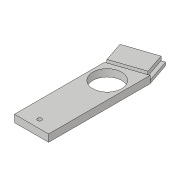
# Autodesk Inventor part: Lidar Sensor Case Piece 2
Saved by Autodesk Inventor 2018.3 (Build 223284000, 284)
## iProperties
Created: 2019-02-26
Part Number: Lidar Sensor Case Piece 2
Material: Generic
Document SubType Name: Modeling
Designer: aye06091
Mass: 11.3761 g
Surface Area: 61.4411 cm^2
Volume: 11.3761 cm^3
Density: 1 g/cm^3
Appearance: Default
Author: aye06091
Autodesk Inventor part; units mm, degrees
ref_plane "YZ Plane" through (0, 0, 0) normal (1, 0, 0) x (0, 1, 0)
ref_plane "XZ Plane" through (0, 0, 0) normal (0, 1, 0) x (-1, 0, 0)
ref_plane "XY Plane" through (0, 0, 0) normal (0, 0, 1) x (1, 0, 0)
sketch "Sketch1" plane through (0, 0, 0) normal (0, 1, 0) x (-1, 0, 0)
  line L0 (18.6455, 5.0782) -> (18.6456, 5.0782)
  line L1 (-34.5212, -28.5033) -> (-28.4641, -46.5646)
  line L2 (-28.4641, -46.5646) -> (-1.974, -37.6808)
  circle A0 centre (-21.2762, -8.5069) radius 11.176
  line L3 (-8.0312, 50.2306) -> (-8.0312, -19.6194)
  line L4 (-8.0312, -19.6194) -> (-1.974, -37.6808)
  line L5 (-1.974, -37.6808) -> (-28.4641, -46.5646)
  line L6 (-28.4641, -46.5646) -> (-34.5212, -28.5033)
  line L7 (-34.5212, -28.5033) -> (-34.5212, 50.2306)
  line L8 (-8.0312, 50.2306) -> (-34.5212, 50.2306)
  point P0 (0, 0)
  dimension "d2" = 27.94
  dimension "d4" = 22.352
  dimension "d24" = 19.05
  dimension "d25" = 69.85
  dimension "d26" = 19.05
  dimension "d28" = 26.49
  dimension "d29" = 13.245
  dimension "d35" = 58.7375
  constraints: 18 end point, 4 perpendicular, 1 centre point, 1 parallel, 1 vertical
  measures "d2" distance of L1.end L2.end
  measures "d4" diameter of A0
  measures "d24" distance of L3.end L2.end
  measures "d25" distance of L3.start L3.end
  measures "d26" distance of L1.start L1.end
  measures "d28" distance of L3.start L7.end
  measures "d29" distance from line of L7 A0.centre
  measures "d35" distance from line of L8 A0.centre
extrude "Extrusion1" add sketch "Sketch1" along normal blind 5.6134
sketch "Sketch2" plane through (0, 5.6134, 0) normal (0, 1, 0) x (1, 0, 0)
  line L0 (34.5212, 28.5034) -> (8.0312, 19.6194)
  line L1 (8.0312, 19.6194) -> (7.0701, 22.4851)
  line L2 (7.0701, 22.4851) -> (33.5601, 31.3691)
  line L3 (31.5176, 27.4961) -> (29.9884, 26.9832)
  line L4 (34.5212, 28.5033) -> (28.4641, 46.5646) projected
  point P0 (0, 0)
  point P1 (0, 0)
  dimension "d11" = 3.0226
  constraints: 8 end point, 4 point on line, 1 parallel, 1 perpendicular
  measures "d11" distance between parallel lines of L2 L0
extrude "Extrusion2" cut sketch "Sketch2" against normal blind 3.175
sketch "Sketch3" plane through (0, 5.6134, 0) normal (0, 1, 0) x (1, 0, 0)
  line L0 (7.0701, 22.4852) -> (33.5601, 31.3691) projected
  line L1 (33.5601, 31.3691) -> (28.4641, 46.5646) projected
  line L2 (28.4641, 46.5646) -> (1.974, 37.6808) projected
  line L3 (25.803, 45.6722) -> (30.8991, 30.4767)
  point P0 (0, 0)
  dimension "d17" = 2.8067
  constraints: 2 end point, 2 point on line, 1 parallel
  measures "d17" distance between parallel lines of L1 L3
extrude "Extrusion3" cut sketch "Sketch3" against normal blind 3.175
sketch "Sketch4" plane through (0, 5.6134, 0) normal (0, 1, 0) x (1, 0, 0)
  line L0 (8.0312, -50.2306) -> (34.5212, -50.2306) projected
  line L1 (34.5212, -50.2306) -> (34.5212, 28.5033) projected
  circle A0 centre (21.2762, -43.8806) radius 1.6002
  point P0 (0, 0)
  dimension "d30" = 3.2004
  dimension "d31" = 13.245
  dimension "d32" = 6.35
  constraints: 1 centre point
  measures "d30" diameter of A0
  measures "d31" distance from line of L1 A0.centre
  measures "d32" distance from line of L0 A0.centre
extrude "Extrusion4" cut sketch "Sketch4" against normal blind 25.4
body "Solid1"
